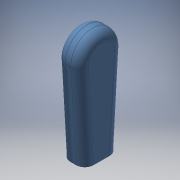
# Autodesk Inventor part: Grip_1
Saved by Autodesk Inventor 2018.1 (Build 221151000, 151)
## iProperties
Created: 2012-05-30
Part Number: Grip_1
Material: Generic
Document SubType Name: Modeling
Designer: normanpa
Density: 1 g/cm^3
Appearance: 127,171,217
Author: normanpa
Autodesk Inventor part; units mm, degrees
ref_plane "YZ Plane" through (0, 0, 0) normal (1, 0, 0) x (0, 1, 0)
ref_plane "XZ Plane" through (0, 0, 0) normal (0, 1, 0) x (-1, 0, 0)
ref_plane "XY Plane" through (0, 0, 0) normal (0, 0, 1) x (1, 0, 0)
sketch "Sketch1" plane through (0, 0, 0) normal (1, 0, 0) x (0, 1, 0)
  line L0 (47.76, 6.35) -> (1.01, 6.35)
  arc A0 (47.76, -6.35) -> (47.76, 6.35) centre (47.76, 0) ccw
  line L1 (1.01, -6.35) -> (47.76, -6.35)
  arc A1 (45.5521, -11.1807) -> (45.5521, 11.1807) centre (46.21, 0) ccw
  line L2 (1.01, 8.56) -> (45.5521, 11.1807)
  line L3 (1.01, -8.56) -> (45.5521, -11.1807)
  line L4 (1.01, 8.56) -> (1.01, -8.56)
  point P0 (0.24, 0)
  point P1 (1.01, 0)
  point P2 (0, 0)
  dimension "d0" = 17.12
  dimension "d2" = 11.2
  dimension "d3" = 2.21
  dimension "d4" = 46.75
  dimension "d5" = 45.2
  dimension "d7" = 8.5
  dimension "d9" = 0.24
  constraints: 10 end point, 4 horizontal alignment, 4 point on circle, 4 tangent, 2 centre point, 2 coincident, 2 point on line, 1 horizontal, 1 midpoint, 1 parallel, 1 perpendicular
  measures "d0" distance of L2.start L3.start
  measures "d2" radius of A1
  measures "d3" distance of L2.start L0.end
  measures "d4" distance of L1.start L1.end
  measures "d5" distance from line of L4 A1.centre
  measures "d7" distance from line of point (0.24, 0) L3
  measures "d9" distance of point (0.24, 0) point (0, 0)
extrude "Extrusion1" add sketch "Sketch1" along normal mid plane 11.8
fillet "Fillet1" radius 4.5 6 edges at (5.9, 57.41, 0) (5.9, 23.281, 9.8703) (5.9, 23.281, -9.8703) (-5.9, 57.41, 0) (-5.9, 23.281, 9.8703) (-5.9, 23.281, -9.8703)
extrude "Extrusion2" cut sketch "Sketch1" along normal mid plane 6.2 contours A0 L1 L4 L0
body "Solid2"
